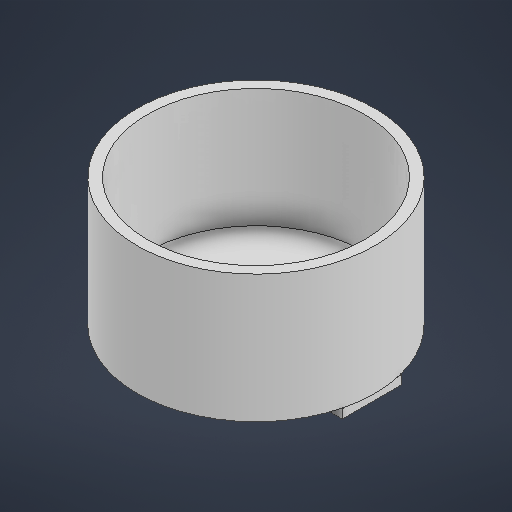
# Autodesk Inventor part: bottomPart
Saved by Autodesk Inventor 2026.2 (Build 302298000, 298)
## iProperties
Created: 2026-04-05
Part Number: bottomPart
Material: Generic
Document SubType Name: Modeling
Designer: Brian Wang
Density: 1 g/cm^3
Appearance: Default
Author: Brian Wang
Autodesk Inventor part; units mm, degrees
ref_plane "YZ Plane" through (0, 0, 0) normal (1, 0, 0) x (0, 1, 0)
ref_plane "XZ Plane" through (0, 0, 0) normal (0, 1, 0) x (-1, 0, 0)
ref_plane "XY Plane" through (0, 0, 0) normal (0, 0, 1) x (1, 0, 0)
sketch "Sketch1" plane through (0, 0, 0) normal (0, 1, 0) x (-1, 0, 0)
  line L0 (39, 10) -> (10, 10)
  line L1 (10, 10) -> (10, 30)
  line L2 (10, 30) -> (-10, 30)
  line L3 (-10, 30) -> (-10, 10)
  line L4 (-10, 10) -> (-39, 10)
  line L5 (-39, 10) -> (-39, -10)
  line L6 (-39, -10) -> (-10, -10)
  line L7 (-10, -10) -> (-10, -30)
  line L8 (-10, -30) -> (10, -30)
  line L9 (10, -30) -> (10, -10)
  line L10 (39, -10) -> (10, -10)
  line L11 (39, -10) -> (39, 10)
  circle A0 centre (25, 5) radius 1.375
  circle A1 centre (-25, 5) radius 1.375
  circle A2 centre (25, -5) radius 1.375
  circle A3 centre (-25, -5) radius 1.375
  point P0 (0, 0)
  dimension "d0" = 29
  dimension "d1" = 20
  dimension "d2" = 90
  dimension "d3" = 20
  dimension "d4" = 90
  dimension "d5" = 29
  dimension "d6" = 20
  dimension "d7" = 90
  dimension "d8" = 20
  dimension "d11" = 2.75
  dimension "d12" = 2.75
  dimension "d13" = 50
  dimension "d14" = 78
  dimension "d15" = 14
  dimension "d16" = 5
  dimension "d20" = 14
  dimension "d21" = 5
  dimension "d22" = 10
  dimension "d23" = 14
  dimension "d24" = 5
  dimension "d25" = 10
  dimension "d26" = 5
  constraints: 24 end point, 8 perpendicular, 8 point on line, 4 centre point, 1 horizontal
  measures "d0" distance of L0.start L0.end
  measures "d1" distance of L0.end L1.end
  measures "d2" angle of L0 L1
  measures "d3" distance of L1.end L2.end
  measures "d4" angle of L2 L1
  measures "d5" distance of L3.end L4.end
  measures "d6" distance of L4.end L5.end
  measures "d7" angle of L5 L4
  measures "d8" distance of L6.end L7.end
  measures "d11" diameter of A0
  measures "d12" diameter of A1
  measures "d13" distance of A1.centre A0.centre
  measures "d14" distance between parallel lines of L11 L5
  measures "d15" distance from line of L11 A0.centre
  measures "d16" distance from line of L0 A0.centre
  measures "d20" distance from line of L11 A2.centre
  measures "d21" distance from line of L10 A2.centre
  measures "d22" distance of A0.centre A2.centre
  measures "d23" distance from line of L5 A3.centre
  measures "d24" distance from line of L6 A3.centre
  measures "d25" distance of A3.centre A1.centre
  measures "d26" distance from line of L4 A1.centre
extrude "Extrusion1" add sketch "Sketch1" along normal blind 3
sketch "Sketch2" plane through (0, 3, 0) normal (0, 1, 0) x (1, 0, 0)
  circle A0 centre (0, 0) radius 40
  dimension "d27" = 80
  constraints: 1 centre point, 1 coincident
  measures "d27" diameter of A0
extrude "Extrusion2" add sketch "Sketch2" along normal blind 3
sketch "Sketch3" plane through (0, 6, 0) normal (0, 1, 0) x (1, 0, 0)
  circle A0 centre (0, 0) radius 40
  circle A1 centre (0, 0) radius 36.5
  dimension "d31" = 73
  constraints: 2 centre point, 2 coincident
  measures "d31" diameter of A1
extrude "Extrusion3" add sketch "Sketch3" along normal blind 40
body "Solid1"
